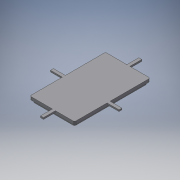
# Autodesk Inventor part: iceTubeClockTop
Saved by Autodesk Inventor 2016 (Build 200138000, 138)
## iProperties
Created: 2016-04-01
Part Number: iceTubeClockTop
Material: Generic
Document SubType Name: Modeling
Designer: boztalay
Density: 1 g/cm^3
Appearance: Default
Author: boztalay
Autodesk Inventor part; units mm, degrees
ref_plane "YZ Plane" through (0, 0, 0) normal (1, 0, 0) x (0, 1, 0)
ref_plane "XZ Plane" through (0, 0, 0) normal (0, 1, 0) x (-1, 0, 0)
ref_plane "XY Plane" through (0, 0, 0) normal (0, 0, 1) x (1, 0, 0)
sketch "Sketch1" plane through (0, 0, 0) normal (0, 1, 0) x (-1, 0, 0)
  line L0 (-44.45, 77.47) -> (44.45, 77.47)
  line L1 (44.45, 77.47) -> (44.45, -77.47)
  line L2 (44.45, -77.47) -> (-44.45, -77.47)
  line L3 (-44.45, -77.47) -> (-44.45, 77.47)
  line L4 (-44.45, 77.47) -> (44.45, -77.47) construction
  line L5 (44.45, 77.47) -> (-44.45, -77.47) construction
  point P0 (0, 0)
  dimension "d0" = 154.94
  dimension "d1" = 88.9
  constraints: 12 end point, 2 midpoint, 2 parallel, 1 horizontal, 1 perpendicular
  measures "d0" distance of L0.end L1.end
  measures "d1" distance of L1.end L2.end
extrude "Extrusion1" add sketch "Sketch1" along normal blind 4.7625
fillet "Fillet1" radius 3.175 4 edges at (44.45, 2.3813, 77.47) (-44.45, 2.3813, 77.47) (44.45, 2.3813, -77.47) (-44.45, 2.3813, -77.47)
sketch "Sketch9" plane through (41.275, 0, -77.47) normal (0, 0, -1) x (-1, 0, 0)
  line L0 (0, 4.7625) -> (82.55, 4.7625) projected
  line L1 (41.275, 0) -> (47.625, 0)
  line L2 (47.625, 0) -> (47.625, 4.7625)
  line L3 (47.625, 4.7625) -> (41.275, 4.7625)
  line L4 (41.275, 4.7625) -> (41.275, 0)
  dimension "d40" = 6.35
  constraints: 8 end point, 2 parallel, 1 horizontal, 1 perpendicular, 1 point on line
  measures "d40" distance of L1.start L1.end
sketch "Sketch10" plane through (-44.45, 0, -74.295) normal (-1, 0, 0) x (0, 0, 1)
  line L0 (0, 4.7625) -> (148.59, 4.7625) projected
  line L1 (74.295, 0) -> (80.645, 0)
  line L2 (80.645, 0) -> (80.645, 4.7625)
  line L3 (80.645, 4.7625) -> (74.295, 4.7625)
  line L4 (74.295, 4.7625) -> (74.295, 0)
  dimension "d41" = 6.35
  constraints: 8 end point, 2 parallel, 1 horizontal, 1 perpendicular, 1 point on line
  measures "d41" distance of L1.start L1.end
sketch "Sketch11" plane through (44.45, 0, 74.295) normal (1, 0, 0) x (0, 0, -1)
  line L0 (148.59, 4.7625) -> (0, 4.7625) projected
  line L1 (74.295, 0) -> (80.645, 0)
  line L2 (80.645, 0) -> (80.645, 4.7625)
  line L3 (80.645, 4.7625) -> (74.295, 4.7625)
  line L4 (74.295, 4.7625) -> (74.295, 0)
  dimension "d42" = 6.35
  constraints: 8 end point, 2 parallel, 1 horizontal, 1 perpendicular, 1 point on line
  measures "d42" distance of L1.start L1.end
sketch "Sketch12" plane through (-41.275, 0, 77.47) normal (0, 0, 1) x (1, 0, 0)
  line L0 (82.55, 4.7625) -> (0, 4.7625) projected
  line L1 (41.275, 0) -> (47.625, 0)
  line L2 (47.625, 0) -> (47.625, 4.7625)
  line L3 (47.625, 4.7625) -> (41.275, 4.7625)
  line L4 (41.275, 4.7625) -> (41.275, 0)
  dimension "d43" = 6.35
  constraints: 8 end point, 2 parallel, 1 horizontal, 1 perpendicular, 1 point on line
  measures "d43" distance of L1.start L1.end
extrude "Extrusion8" add sketch "Sketch11" along normal blind 25.4
extrude "Extrusion9" add sketch "Sketch12" along normal blind 25.4
extrude "Extrusion10" add sketch "Sketch10" along normal blind 25.4
extrude "Extrusion11" add sketch "Sketch9" along normal blind 25.4
body "Solid1"
